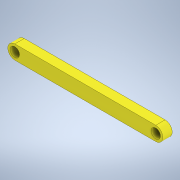
# Autodesk Inventor part: outerLink
Saved by Autodesk Inventor 2022 (Build 260153000, 153)
## iProperties
Created: 2021-12-27
Part Number: outerLink
Material: Generic
Document SubType Name: Modeling
Designer: G S SHOURIE
Density: 1 g/cm^3
Appearance: Canary
Author: G S SHOURIE
Autodesk Inventor part; units mm, degrees
ref_plane "YZ Plane" through (0, 0, 0) normal (1, 0, 0) x (0, 1, 0)
ref_plane "XZ Plane" through (0, 0, 0) normal (0, 1, 0) x (-1, 0, 0)
ref_plane "XY Plane" through (0, 0, 0) normal (0, 0, 1) x (1, 0, 0)
sketch "Sketch2" plane through (0, 0, 0) normal (0, 0, 1) x (1, 0, 0)
  line L0 (-37.5, 7.5) -> (112.5, 7.5)
  line L1 (112.5, 7.5) -> (112.5, -7.5)
  line L2 (112.5, -7.5) -> (-37.5, -7.5)
  line L3 (-37.5, -7.5) -> (-37.5, 7.5)
  arc A0 (-37.5, 7.5) -> (-37.5, -7.5) centre (-37.5, 0) ccw
  arc A1 (112.5, -7.5) -> (112.5, 7.5) centre (112.5, 0) ccw
  circle A2 centre (-37.5, 0) radius 5
  circle A3 centre (36.6347, 0) radius 5
  point P0 (0, 0)
  point P1 (-37.5, 5)
  point P2 (-37.5, -5)
  dimension "d8" = 150
  dimension "d9" = 15
  dimension "d10" = 7.5
  dimension "d11" = 37.5
  dimension "d12" = 10
  dimension "d13" = 10
  constraints: 8 end point, 4 centre point, 4 point on circle, 2 midpoint, 2 parallel, 1 coincident, 1 horizontal, 1 perpendicular
  measures "d8" distance of L1.end L2.end
  measures "d9" distance of L0.end L1.end
  measures "d10" distance from line of L0 point (0, 0)
  measures "d11" distance from line of L3 point (0, 0)
  measures "d12" diameter of A2
  measures "d13" diameter of A3
extrude "Extrusion2" add sketch "Sketch2" along normal blind 10 contours L0 L1 L2 L3 A2 | L3 A2 A0 | A1 L1 | A2 L3 | L3 A2 | A3
sketch "Sketch3" plane through (0, 0, 10) normal (0, 0, 1) x (1, 0, 0)
  circle A0 centre (-37.5, 0) radius 5
  arc A1 (112.5, -7.5) -> (112.5, 7.5) centre (112.5, 0) ccw projected
  circle A2 centre (112.5, 0) radius 5
  point P0 (0, 0)
  dimension "d16" = 10
  dimension "d17" = 10
  constraints: 2 centre point, 1 coincident
  measures "d16" diameter of A0
  measures "d17" diameter of A2
extrude "Extrusion3" cut sketch "Sketch3" against normal blind 10
body "Solid2"
